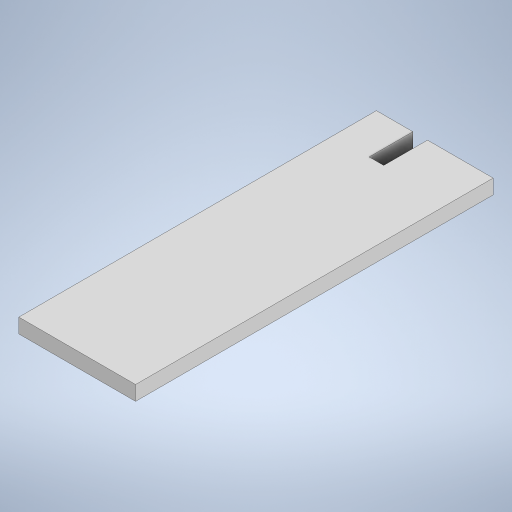
# Autodesk Inventor part: back_1
Saved by Autodesk Inventor 2023 (Build 270158000, 158)
## iProperties
Created: 2024-04-26
Part Number: back_1
Material: 常规
Document SubType Name: Modeling
Designer: Nitrene.P.L
Density: 1 g/cm^3
Appearance: 默认
Author: Nitrene.P.L
Autodesk Inventor part; units mm, degrees
ref_plane "YZ Plane" through (0, 0, 0) normal (1, 0, 0) x (0, 1, 0)
ref_plane "XZ Plane" through (0, 0, 0) normal (0, 1, 0) x (-1, 0, 0)
ref_plane "XY Plane" through (0, 0, 0) normal (0, 0, 1) x (1, 0, 0)
sketch "草图1" plane through (0, 0, 0) normal (0, 1, 0) x (-1, 0, 0)
  line L0 (40, 245) -> (-40, 245)
  line L1 (-40, 245) -> (-40, -245)
  line L2 (-40, -245) -> (40, -245)
  line L3 (40, -245) -> (40, 245)
  line L4 (0, 5.532) -> (0, -5.7915)
  line L5 (3, 0) -> (-2, 0)
  line L6 (40, 0) -> (-40, 0)
  line L7 (15, 30) -> (5, 30)
  line L8 (5, 30) -> (5, -30)
  line L9 (5, -30) -> (15, -30)
  line L10 (15, -30) -> (15, 30)
  point P0 (0, 0)
  point P1 (0, 0)
  point P2 (0, 0)
  point P3 (-2, 0)
  point P4 (5, 0)
  point P5 (15, 0)
  dimension "d0" = 80
  dimension "d1" = 490
  dimension "d2" = 10
  dimension "d3" = 60
  dimension "d4" = 25
  constraints: 22 end point, 4 parallel, 3 horizontal, 2 midpoint, 2 perpendicular, 2 vertical, 3 other
  measures "d0" distance of L2.end L1.end
  measures "d1" distance of L1.end L0.end
  measures "d2" distance of L9.end L8.end
  measures "d3" distance of L8.end L7.end
  measures "d4" distance between parallel lines of L3 L10
extrude "拉伸1" add sketch "草图1" along normal blind 10 contours L3 L6 L10 L7 L8 L5 L1 L0
